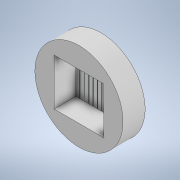
# Autodesk Inventor part: FDMPrintHeadPlanarPrototypes
Saved by Autodesk Inventor 2021 (Build 250183000, 183)
## iProperties
Created: 2022-02-04
Part Number: FDMPrintHeadPlanarPrototypes
Material: Generic
Document SubType Name: Sheet Metal
Designer: Unit-005
Density: 1 g/cm^3
Sheet Metal Rule: Default
Appearance: Default
Author: Unit-005
## iProperties of the stored document _3DPrint.ipt
Created: 2022-02-04
Part Number: _3DPrint
Material: Generic
Document SubType Name: Modeling
Designer: Unit-005
Density: 1 g/cm^3
Appearance: Default
Author: Unit-005
Autodesk Inventor part; units mm, degrees
ref_plane "YZ Plane" through (0, 0, 0) normal (1, 0, 0) x (0, 1, 0)
ref_plane "XZ Plane" through (0, 0, 0) normal (0, 1, 0) x (-1, 0, 0)
ref_plane "XY Plane" through (0, 0, 0) normal (0, 0, 1) x (1, 0, 0)
sketch "Sketch1" plane through (0, 0, 0) normal (0, 0, 1) x (1, 0, 0)
  line L0 (-14.3446, 13.462) -> (14.3446, 13.462)
  line L1 (14.3446, 13.462) -> (14.3446, -13.462)
  line L2 (14.3446, -13.462) -> (-14.3446, -13.462)
  line L3 (-14.3446, -13.462) -> (-14.3446, 13.462)
  line L4 (-14.3446, 13.462) -> (14.3446, -13.462) construction
  line L5 (14.3446, 13.462) -> (-14.3446, -13.462) construction
  point P0 (0, 0)
  dimension "d0" = 28.6893
  dimension "d1" = 26.924
  constraints: 12 end point, 2 midpoint, 2 parallel, 1 horizontal, 1 perpendicular
  measures "d0" distance of L1.end L2.end
  measures "d1" distance of L0.end L1.end
ref_plane "Work Plane1" through (0, 0, 0) normal (0, 0, -1) x (-1, 0, 0)
sketch "Sketch2" plane through (0, 0, 0) normal (0, 0, -1) x (-1, 0, 0)
  circle A0 centre (0, 0) radius 25.4
  dimension "d4" = 50.8
  constraints: 1 centre point, 1 coincident
  measures "d4" diameter of A0
extrude "Extrusion2" add sketch "Sketch2" against normal blind 12.7
extrude "Extrusion3" cut sketch "Sketch1" along normal through all
sketch "Sketch3" plane through (0, 0, 0) normal (0, 0, 1) x (1, 0, 0)
  line L0 (-14.3446, -13.462) -> (14.3446, -13.462) projected
  line L1 (-14.3446, 13.462) -> (-14.3446, -13.462) projected
  line L2 (14.3446, 13.462) -> (-14.3446, 13.462) projected
  line L3 (14.3446, -13.462) -> (14.3446, 13.462) projected
  line L4 (-14.3446, 13.462) -> (-14.3446, -13.462) projected
  line L5 (-14.3446, -13.462) -> (14.3446, -13.462) projected
  line L6 (14.3446, -13.462) -> (14.3446, 13.462) projected
  line L7 (14.3446, 13.462) -> (-14.3446, 13.462) projected
  circle A0 centre (0, 0) radius 25.4 projected
  line L8 (-35.56, 0) -> (35.56, 0) projected
  line L9 (0, -35.56) -> (0, 35.56) projected
  line L10 (14.3446, 13.462) -> (-14.3446, 13.462) projected
  line L11 (-14.3446, -13.462) -> (14.3446, -13.462)
  line L12 (14.3446, -13.462) -> (14.3446, 13.462)
  line L13 (14.3446, 13.462) -> (-14.3446, 13.462)
  line L14 (-14.3446, 13.462) -> (-14.3446, -13.462)
  line L15 (-14.3446, -13.462) -> (14.3446, 13.462) construction
  line L16 (14.3446, -13.462) -> (-14.3446, 13.462) construction
  line L17 (14.3446, 13.462) -> (-14.3446, 13.462) projected
  line L18 (-14.3446, -13.462) -> (-12.1856, -13.462)
  line L19 (-12.1856, -13.462) -> (-12.1856, 13.462)
  line L20 (-12.1856, 13.462) -> (-14.3446, 13.462)
  line L21 (-14.3446, 13.462) -> (-14.3446, -13.462)
  line L22 (-14.3446, -13.462) -> (-12.1856, 13.462) construction
  line L23 (-12.1856, -13.462) -> (-14.3446, 13.462) construction
  point P0 (-13.2651, 0)
  dimension "d9" = 2.159
  constraints: 24 end point, 4 midpoint, 4 parallel, 2 collinear, 2 horizontal, 2 perpendicular, 2 point on line
  measures "d9" distance of L20.end L19.end
extrude "Extrusion4" add sketch "Sketch3" along normal blind 0.1524 contours L1 L8 L19 L0 | L1 L2 L19 L8
pattern_linear "Rectangular Pattern1" count 12 spacing 2.54 along (1, 0, 0) of "Extrusion4"
sketch "Sketch4" plane through (0, 0, 0) normal (0, 0, 1) x (1, 0, 0)
  line L0 (13.2144, -13.462) -> (13.5954, -13.462) projected
  line L1 (13.5954, 13.462) -> (13.5954, -13.462) projected
  line L2 (13.5954, 13.462) -> (13.2144, 13.462) projected
  line L3 (13.2144, -13.462) -> (13.2144, 13.462) projected
  line L4 (11.0554, 13.462) -> (11.0554, -13.462) projected
  line L5 (11.0554, 13.462) -> (10.6744, 13.462) projected
  line L6 (10.6744, -13.462) -> (10.6744, 13.462) projected
  line L7 (10.6744, -13.462) -> (11.0554, -13.462) projected
  line L8 (8.5154, 13.462) -> (8.5154, -13.462) projected
  line L9 (8.5154, 13.462) -> (8.1344, 13.462) projected
  line L10 (8.1344, -13.462) -> (8.1344, 13.462) projected
  line L11 (8.1344, -13.462) -> (8.5154, -13.462) projected
  line L12 (5.9754, 13.462) -> (5.9754, -13.462) projected
  line L13 (5.9754, 13.462) -> (5.5944, 13.462) projected
  line L14 (5.5944, -13.462) -> (5.5944, 13.462) projected
  line L15 (5.5944, -13.462) -> (5.9754, -13.462) projected
  line L16 (3.4354, 13.462) -> (3.4354, -13.462) projected
  line L17 (3.4354, 13.462) -> (3.0544, 13.462) projected
  line L18 (3.0544, -13.462) -> (3.0544, 13.462) projected
  line L19 (3.0544, -13.462) -> (3.4354, -13.462) projected
  line L20 (0.8954, 13.462) -> (0.8954, -13.462) projected
  line L21 (0.8954, 13.462) -> (0.5144, 13.462) projected
  line L22 (0.5144, -13.462) -> (0.5144, 13.462) projected
  line L23 (0.5144, -13.462) -> (0.8954, -13.462) projected
  line L24 (-1.6446, 13.462) -> (-1.6446, -13.462) projected
  line L25 (-1.6446, 13.462) -> (-2.0256, 13.462) projected
  line L26 (-2.0256, -13.462) -> (-2.0256, 13.462) projected
  line L27 (-2.0256, -13.462) -> (-1.6446, -13.462) projected
  line L28 (-4.1846, 13.462) -> (-4.1846, -13.462) projected
  line L29 (-4.1846, 13.462) -> (-4.5656, 13.462) projected
  line L30 (-4.5656, -13.462) -> (-4.5656, 13.462) projected
  line L31 (-4.5656, -13.462) -> (-4.1846, -13.462) projected
  line L32 (-6.7246, 13.462) -> (-6.7246, -13.462) projected
  line L33 (-6.7246, 13.462) -> (-7.1056, 13.462) projected
  line L34 (-7.1056, -13.462) -> (-7.1056, 13.462) projected
  line L35 (-7.1056, -13.462) -> (-6.7246, -13.462) projected
  line L36 (-9.2646, 13.462) -> (-9.2646, -13.462) projected
  line L37 (-9.2646, 13.462) -> (-9.6456, 13.462) projected
  line L38 (-9.6456, -13.462) -> (-9.6456, 13.462) projected
  line L39 (-9.6456, -13.462) -> (-9.2646, -13.462) projected
  circle A0 centre (0, 0) radius 25.4 projected
  line L40 (-11.8046, 13.462) -> (-11.8046, -13.462) projected
  line L41 (-11.8046, 13.462) -> (-12.1856, 13.462) projected
  line L42 (-12.1856, -13.462) -> (-12.1856, 13.462) projected
  line L43 (-12.1856, -13.462) -> (-11.8046, -13.462) projected
  line L44 (-35.56, 0) -> (35.56, 0) projected
  line L45 (0, -35.56) -> (0, 35.56) projected
  line L46 (-12.1856, -13.462) -> (-11.8046, -13.462) projected
  line L47 (13.5954, 13.462) -> (13.5954, -13.462) projected
  line L48 (-12.1856, -13.462) -> (13.5954, -13.462)
  line L49 (13.5954, -13.462) -> (13.5954, -0.254)
  line L50 (13.5954, -0.254) -> (-12.1857, -0.254)
  line L51 (-12.1857, -0.254) -> (-12.1856, -13.462)
  line L52 (13.2144, 13.462) -> (13.5954, 13.462)
  line L53 (10.6744, 13.462) -> (11.0554, 13.462)
  line L54 (8.1344, 13.462) -> (8.5154, 13.462)
  line L55 (5.5944, 13.462) -> (5.9754, 13.462)
  line L56 (3.0544, 13.462) -> (3.4354, 13.462)
  line L57 (0.5144, 13.462) -> (0.8954, 13.462)
  line L58 (-2.0256, 13.462) -> (-1.6446, 13.462)
  line L59 (-4.5656, 13.462) -> (-4.1846, 13.462)
  line L60 (-7.1056, 13.462) -> (-6.7246, 13.462)
  line L61 (-9.6456, 13.462) -> (-9.2646, 13.462)
  line L62 (-12.1856, 13.462) -> (-11.8046, 13.462)
  line L63 (-12.1856, 13.462) -> (-11.8046, 13.462)
  line L64 (-12.1856, 13.462) -> (13.5954, 13.462)
  line L65 (13.5954, 13.462) -> (13.5954, 0.254)
  line L66 (13.5954, 0.254) -> (-12.1857, 0.254)
  line L67 (-12.1857, 0.254) -> (-12.1856, 13.462)
  dimension "d15" = 0.254
  constraints: 36 end point, 4 symmetric about line, 1 horizontal, 1 parallel, 1 point on line, 1 vertical, 6 other
  measures "d15" distance between parallel lines of L44 L50
extrude "Extrusion5" [suppressed]
sketch "Sketch5" plane through (0, 0, 0) normal (0, 0, -1) x (-1, 0, 0)
  line L0 (-13.2144, -13.462) -> (-13.2144, 13.462) projected
  line L1 (-13.5954, 13.462) -> (-13.5954, -13.462) projected
  line L2 (-10.6744, -13.462) -> (-10.6744, 13.462) projected
  line L3 (-11.0554, 13.462) -> (-11.0554, -13.462) projected
  line L4 (-8.1344, -13.462) -> (-8.1344, 13.462) projected
  line L5 (-8.5154, 13.462) -> (-8.5154, -13.462) projected
  line L6 (-5.5944, -13.462) -> (-5.5944, 13.462) projected
  line L7 (-5.9754, 13.462) -> (-5.9754, -13.462) projected
  line L8 (-3.0544, -13.462) -> (-3.0544, 13.462) projected
  line L9 (-3.4354, 13.462) -> (-3.4354, -13.462) projected
  line L10 (-0.5144, -13.462) -> (-0.5144, 13.462) projected
  line L11 (-0.8954, 13.462) -> (-0.8954, -13.462) projected
  line L12 (2.0256, -13.462) -> (2.0256, 13.462) projected
  line L13 (1.6446, 13.462) -> (1.6446, -13.462) projected
  line L14 (4.5656, -13.462) -> (4.5656, 13.462) projected
  line L15 (4.1846, 13.462) -> (4.1846, -13.462) projected
  line L16 (7.1056, -13.462) -> (7.1056, 13.462) projected
  line L17 (6.7246, 13.462) -> (6.7246, -13.462) projected
  line L18 (9.6456, -13.462) -> (9.6456, 13.462) projected
  line L19 (9.2646, 13.462) -> (9.2646, -13.462) projected
  circle A0 centre (0, 0) radius 25.4 projected
  line L20 (12.1856, -13.462) -> (12.1856, 13.462) projected
  line L21 (11.8046, 13.462) -> (11.8046, -13.462) projected
  line L22 (35.56, 0) -> (-35.56, 0) projected
  line L23 (0, -35.56) -> (0, 35.56) projected
  circle A1 centre (11.9952, -2.794) radius 0.5
  line L24 (-13.2144, -13.462) -> (-13.5954, -13.462) projected
  line L25 (-13.5954, 13.462) -> (-13.2144, 13.462) projected
  line L26 (-11.0554, 13.462) -> (-10.6744, 13.462) projected
  line L27 (-10.6744, -13.462) -> (-11.0554, -13.462) projected
  line L28 (-8.5154, 13.462) -> (-8.1344, 13.462) projected
  line L29 (-8.1344, -13.462) -> (-8.5154, -13.462) projected
  line L30 (-5.9754, 13.462) -> (-5.5944, 13.462) projected
  line L31 (-5.5944, -13.462) -> (-5.9754, -13.462) projected
  line L32 (-3.4354, 13.462) -> (-3.0544, 13.462) projected
  line L33 (-3.0544, -13.462) -> (-3.4354, -13.462) projected
  line L34 (-0.8954, 13.462) -> (-0.5144, 13.462) projected
  line L35 (-0.5144, -13.462) -> (-0.8954, -13.462) projected
  line L36 (1.6446, 13.462) -> (2.0256, 13.462) projected
  line L37 (2.0256, -13.462) -> (1.6446, -13.462) projected
  line L38 (4.1846, 13.462) -> (4.5656, 13.462) projected
  line L39 (4.5656, -13.462) -> (4.1846, -13.462) projected
  line L40 (6.7246, 13.462) -> (7.1056, 13.462) projected
  line L41 (7.1056, -13.462) -> (6.7246, -13.462) projected
  line L42 (9.2646, 13.462) -> (9.6456, 13.462) projected
  line L43 (9.6456, -13.462) -> (9.2646, -13.462) projected
  line L44 (11.8046, 13.462) -> (12.1856, 13.462) projected
  line L45 (12.1856, -13.462) -> (11.8046, -13.462) projected
  point P0 (11.9952, -0.254)
  dimension "d18" = 1
  constraints: 1 centre point, 1 vertical alignment
  measures "d18" diameter of A1
extrude "Extrusion6" [suppressed]
pattern_linear "Rectangular Pattern2" [suppressed]
mirror "Mirror1" [suppressed]
equation "\"BendRadius\" = Thickness"
equation "\"BendReliefWidth\" = Thickness"
equation "\"BendReliefDepth\" = 0.5 * Thickness"
equation "\"CornerReliefSize\" = 4 * Thickness"
equation "\"MinimumRemnant\" = 2 * Thickness"
equation "\"TransitionRadius\" = BendRadius"
equation "\"JacobiRadiusSize\" = BendRadius"
equation "\"GapSize\" = Thickness"
equation "\"Thickness\" = 3.048"
body "Solid2"
